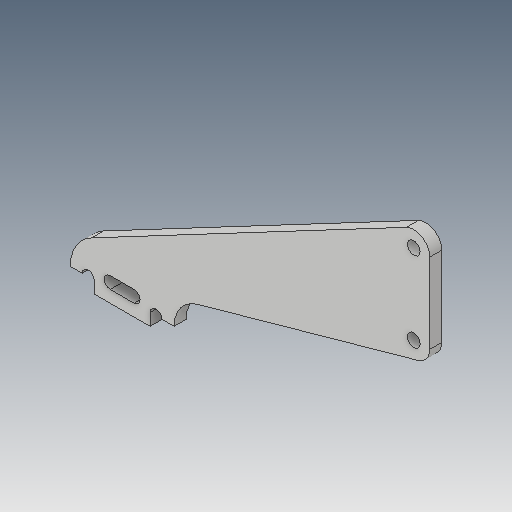
# Autodesk Inventor part: BaseSliderSupport
Saved by Autodesk Inventor 2019.4 (Build 234330000, 330)
## iProperties
Created: 2019-07-01
Part Number: BaseSliderSupport
Material: Generic
Document SubType Name: Modeling
Designer: AzLIer
Density: 1 g/cm^3
Appearance: Default
Author: AzLIer
Autodesk Inventor part; units mm, degrees
ref_plane "YZ Plane" through (0, 0, 0) normal (1, 0, 0) x (0, 1, 0)
ref_plane "XZ Plane" through (0, 0, 0) normal (0, 1, 0) x (-1, 0, 0)
ref_plane "XY Plane" through (0, 0, 0) normal (0, 0, 1) x (1, 0, 0)
sketch "スケッチ1" plane through (0, 0, 0) normal (0, 0, 1) x (1, 0, 0)
  line L0 (1.0771, -3.8522) -> (-54.1543, -19.2955)
  line L1 (-60, -27) -> (-63, -27)
  arc A0 (-63, -27) -> (-66, -27) centre (-64.5, -27) ccw
  line L2 (-66, -27) -> (-66, -30)
  line L3 (-66, -30) -> (-80, -30)
  line L4 (-80, -30) -> (-80, -27)
  arc A1 (-80, -27) -> (-83, -27) centre (-81.5, -27) ccw
  line L5 (-83, -27) -> (-86, -27)
  arc A2 (-80.6768, -18.161) -> (-86, -27) centre (-76, -27) ccw
  line L6 (-80.6768, -18.161) -> (-1.8707, 23.5356)
  line L7 (4, 20) -> (4, 0)
  line L8 (-76, -25.5) -> (-70, -25.5) construction
  line L9 (-76, -27) -> (-70, -27)
  line L10 (-70, -24) -> (-76, -24)
  arc A3 (-76, -24) -> (-76, -27) centre (-76, -25.5) ccw
  arc A4 (-70, -27) -> (-70, -24) centre (-70, -25.5) ccw
  circle A5 centre (0, 0) radius 1.6
  circle A6 centre (0, 20) radius 1.6
  arc A7 (1.0771, -3.8522) -> (4, 0) centre (0, 0) ccw
  arc A8 (4, 20) -> (-1.8707, 23.5356) centre (0, 20) ccw
  arc A9 (-54.1543, -19.2955) -> (-60, -27) centre (-52, -27) ccw
  point P0 (-73, -25.5)
  point P1 (-73, -30)
  dimension "d0" = 3
  dimension "d1" = 6
  dimension "d2" = 14
  dimension "d3" = 1.5
  dimension "d4" = 3
  dimension "d5" = 1.5
  dimension "d6" = 3
  dimension "d9" = 3.2
  dimension "d10" = 3.2
  dimension "d13" = 4
  dimension "d14" = 20
  dimension "d15" = 30
  dimension "d16" = 10
  dimension "d19" = 8
  dimension "d20" = 60
  constraints: 24 end point, 16 point on circle, 12 tangent, 10 centre point, 5 point on line, 3 horizontal, 3 perpendicular, 2 coincident, 2 equal radius, 2 midpoint, 2 vertical alignment, 1 collinear, 1 line through centre, 1 parallel, 1 vertical, 1 other
  measures "d0" distance of L3.end L4.end
  measures "d1" distance of L8.start L8.end
  measures "d2" distance of L2.end L3.end
  measures "d3" radius of A0
  measures "d4" distance of L1.start L1.end
  measures "d5" radius of A3
  measures "d6" distance between parallel lines of L3 L9
  measures "d9" diameter of A5
  measures "d10" diameter of A6
  measures "d13" radius of A7
  measures "d14" distance of A6.centre A5.centre
  measures "d15" distance from line of A5.centre L3
  measures "d16" radius of A2
  measures "d19" radius of A9
  measures "d20" horizontal distance of A5.centre L1.start
extrude "押し出し1" add sketch "スケッチ1" along normal blind 3
equation "\"d6\" = d0"
